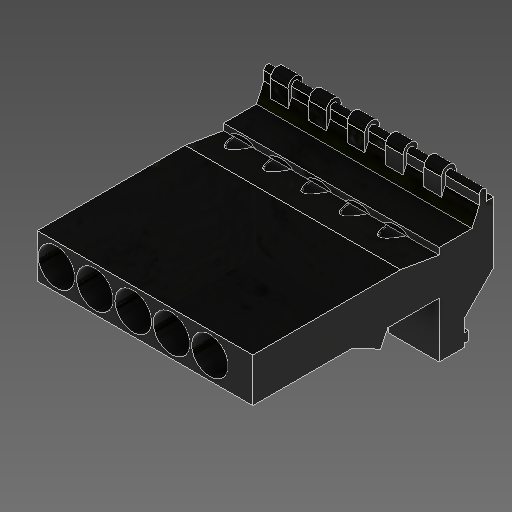
# Autodesk Inventor part: PostValveLast0
Saved by Autodesk Inventor 2020 (Build 240168000, 168)
## iProperties
Created: 2018-10-10
Part Number: PostValveLast0
Material: PLA Plastic (Black)
Document SubType Name: Modeling
Designer: Isaac Newcomb
Density: 1.06 g/cm^3
Appearance: 3D Printed - Black
Mass: 35.4889 g
Surface Area: 271.602 cm^2
Volume: 33.4801 cm^3
HingeHeight: 7.000 mm
KeyWidth: 10.000 mm
WhistleHousingHeight: 12.000 mm
PVBoxHeight: 20.163 mm
WhistleHousingLength: 51.000 mm
PVBoxDepth: 15.000 mm
HingeRadius: 1.000 mm
HingeOffset: 2.000 mm
HingeBigRadius: 2.000 mm
HingeBlockHeight: 4.500 mm
TubeSocketLength: 10.000 mm
SiliconeFittingLength: 10.000 mm
KeyCount: 25.000 ul
KeySpacing: 0.500 mm
SpringBlockHeight: 7.000 mm
SpringPassChamferLength: 8.000 mm
PincherTriangleHeight: 4.081 mm
PincherTriangleOffset: 31.000 mm
ManifoldWidth: 15.000 mm
ManifoldFittingLength: 10.000 mm
WhistleHousingVertWallThickness: 1.400 mm
Author: Isaac Newcomb
Autodesk Inventor part; units mm, degrees
ref_plane "YZ Plane" through (0, 0, 0) normal (1, 0, 0) x (0, 1, 0)
ref_plane "XZ Plane" through (0, 0, 0) normal (0, 1, 0) x (-1, 0, 0)
ref_plane "XY Plane" through (0, 0, 0) normal (0, 0, 1) x (1, 0, 0)
sketch "Base Sketch" plane through (0, 0, 0) normal (0, 0, 1) x (1, 0, 0)
  line L0 (0, 0) -> (10.5, 0)
  line L1 (10.5, 0) -> (10.5, 20.1625)
  line L2 (10.5, 20.1625) -> (0, 20.1625)
  line L3 (0, 20.1625) -> (0, 0)
  line L4 (1, 19.1625) -> (9.5, 19.1625)
  line L5 (9.5, 19.1625) -> (9.5, 1)
  line L6 (9.5, 1) -> (1, 1)
  line L7 (1, 1) -> (1, 19.1625)
  dimension "PVBoxWidth" = 10.5
  dimension "PVBoxHeight" = 20.1625
  dimension "SideWallThickness" = 1
  constraints: 16 end point, 4 parallel, 2 perpendicular, 1 horizontal, 3 other
  measures "PVBoxWidth" distance of L2.end L1.end
  measures "PVBoxHeight" distance of L2.end L0.start
  measures "SideWallThickness" distance between parallel lines of L2 L4
extrude "Side Walls" add sketch "Base Sketch" along normal blind 15
extrude "Back Wall" add sketch "Base Sketch" along normal blind 1 contours L4 L5 L6 L7
sketch "Sketch5" plane through (0, 0, 15) normal (0, 0, 1) x (1, 0, 0)
  line L0 (1, 19.1625) -> (9.5, 19.1625) projected
  line L1 (1, 1) -> (1, 19.1625) projected
  line L2 (9.5, 1) -> (1, 1) projected
  line L3 (9.5, 19.1625) -> (9.5, 1) projected
  point P0 (0, 0)
extrude "Front Wall" add sketch "Sketch5" against normal blind 5
sketch "Whistle Housing Sketch" plane through (0, 0, 15) normal (0, 0, 1) x (1, 0, 0)
  line L0 (0, 0) -> (10.5, 0) projected
  line L1 (0, 0) -> (0, 12)
  line L2 (0, 12) -> (10.5, 12)
  line L3 (10.5, 12) -> (10.5, 0)
  circle A0 centre (5.25, 6) radius 4.6
  line L4 (0, 6) -> (10.5, 6) construction
  line L5 (0, 12) -> (10.5, 12)
  line L6 (10.5, 12) -> (10.5, 15.5)
  line L7 (10.5, 15.5) -> (0, 15.5)
  line L8 (0, 15.5) -> (0, 12)
  dimension "WhistleHousingHeight" = 12
  dimension "TubeInnerDiameter" = 9.2
  dimension "TabThickness" = 3.5
  constraints: 16 end point, 3 midpoint, 3 perpendicular, 2 parallel, 1 centre point, 1 coincident, 1 horizontal, 1 vertical
  measures "WhistleHousingHeight" distance of L0.start L1.end
  measures "TubeInnerDiameter" diameter of A0
  measures "TabThickness" distance of L7.end L1.end
extrude "Whistle Housing" add sketch "Whistle Housing Sketch" along normal blind 51 contours L1 L2 L3 L0
sketch "Tube Socket Sketch" plane through (0, 0, 66) normal (0, 0, 1) x (1, 0, 0)
  circle A0 centre (5.25, 6) radius 4.6 construction
  circle A1 centre (5.25, 6) radius 5
  point P0 (0, 0)
  dimension "d78" = 10
  constraints: 1 centre point, 1 coincident
  measures "d78" diameter of A1
extrude "Tube Socket" cut sketch "Tube Socket Sketch" against normal blind 10
ref_plane "Midplane" through (5.25, 0, 0) normal (1, 0, 0) x (0, 0, -1)
sketch "Slit Sketch" plane through (0, 0, 15) normal (0, 0, 1) x (1, 0, 0)
  arc A0 (1.6989, 1.8) -> (8.8011, 1.8) centre (5.25, 6) ccw
  line L0 (8.8011, 1.8) -> (1.6989, 1.8)
  point P0 (0, 0)
  dimension "d81" = 11
  dimension "d187" = 5.25
  dimension "d188" = 6
  dimension "d193" = 4.2
  dimension "d194" = 1.3
  constraints: 2 end point, 2 point on circle, 1 centre point, 1 horizontal
  measures "d81" diameter of A0
  measures "d187" horizontal distance of point (0, 0) A0.centre
  measures "d188" vertical distance of point (0, 0) A0.centre
  measures "d193" distance from line of L0 A0.centre
  measures "d194" distance edge to line of A0 L0
extrude "Slit" cut sketch "Slit Sketch" against normal up to surface (14 mm away)
sketch "Silicone Fitting Sketch" plane through (5.25, 0, 0) normal (1, 0, 0) x (0, 0, -1)
  line L0 (-15, 20.1625) -> (-15, 12) projected
  line L1 (-15, 16.0813) -> (-25, 16.0813) construction
  line L2 (-25, 16.0813) -> (-25, 18.4625)
  line L3 (-25, 18.4625) -> (-22, 18.4625) construction
  line L4 (-25, 18.4625) -> (-22, 19.1625)
  line L5 (-22, 19.1625) -> (-22, 18.4625)
  line L6 (-25, 17.9625) -> (-15, 17.9625)
  line L7 (-22, 18.4625) -> (-19, 18.4625) construction
  line L8 (-15, 19.1625) -> (-22, 19.1625) construction
  line L9 (-22, 18.4625) -> (-19, 19.1625)
  line L10 (-19, 19.1625) -> (-19, 18.4625)
  line L11 (-19, 18.4625) -> (-15, 18.4625)
  point P0 (0, 0)
  point P1 (-15, 0)
  dimension "SiliconeFittingLength" = 10
  dimension "d65" = 2.3813
  dimension "d66" = 3
  dimension "d67" = 0.7
  dimension "d68" = 0.5
  constraints: 22 end point, 10 perpendicular, 5 point on line, 4 parallel, 2 horizontal, 2 midpoint
  measures "SiliconeFittingLength" distance of L1.start L1.end
  measures "d65" distance of L1.end L2.end
  measures "d66" horizontal distance of L4.end L2.end
  measures "d67" distance of L4.end L3.end
  measures "d68" distance between parallel lines of L3 L6
revolve "Silicone Fitting" add sketch "Silicone Fitting Sketch" angle 360 about axis through (5.25, 16.0813, 15) along (0, 0, 1)
sketch "Silicone Fitting to Chamber Sketch" plane through (5.25, 16.0813, 15) normal (0, 0, 1) x (1, 0, 0)
  circle A0 centre (0, 0) radius 1.8813 projected
  point P0 (-5.25, -16.0813)
extrude "Silicone Fitting to Chamber" cut sketch "Silicone Fitting to Chamber Sketch" against normal up to surface (5 mm away)
sketch "Hinge Sketch" plane through (10.5, 0, 0) normal (1, 0, 0) x (0, 0, -1)
  line L0 (0, 0) -> (-66, 0) projected
  line L1 (-2, 0) -> (-2, -4.5) construction
  arc A0 (-4, -7) -> (-2, -7) centre (-3, -7) ccw
  line L2 (-4, -7) -> (-4, -4.5)
  line L3 (-2, -4.5) -> (0, -4.5)
  line L4 (0, -4.5) -> (0, 0)
  line L5 (-4, -4.5) -> (-6, -4.5)
  line L6 (-6, -4.5) -> (-6, 0)
  line L7 (-2, -4.5) -> (-2, -7)
  line L8 (-4, -4.5) -> (-4, 0) construction
  point P0 (-15, 0)
  dimension "HingeRadius" = 1
  dimension "HingeBlockHeight" = 4.5
  dimension "HingeOffset" = 2
  dimension "HingeHeight" = 7
  constraints: 16 end point, 5 point on line, 4 perpendicular, 4 tangent, 2 point on circle, 2 vertical, 1 centre point, 1 collinear, 1 horizontal
  measures "HingeRadius" radius of A0
  measures "HingeBlockHeight" distance of L3.end L0.start
  measures "HingeOffset" distance of L1.end L3.end
  measures "HingeHeight" distance from line of L0 A0.centre
extrude "Hinge" add sketch "Hinge Sketch" against normal blind 10.5
sketch "Hinge Nub Sketch" plane through (5.25, 20.1625, 15) normal (1, 0, 0) x (0, 0, -1)
  arc A0 (11, -27.1625) -> (13, -27.1625) centre (12, -27.1625) ccw construction
  arc A1 (10, -27.1625) -> (14, -27.1625) centre (12, -27.1625) ccw
  line L0 (14, -27.1625) -> (14, -24.6625)
  line L1 (15, -24.6625) -> (9, -24.6625)
  line L2 (10, -24.6625) -> (10, -27.1625)
  point P0 (15, -20.1625)
  point P1 (9, -20.1625)
  dimension "HingeBigRadius" = 2
  constraints: 6 end point, 2 point on circle, 2 point on line, 2 tangent, 1 centre point, 1 coincident, 1 parallel, 1 perpendicular, 1 vertical
  measures "HingeBigRadius" radius of A1
extrude "Hinge Nub" add sketch "Hinge Nub Sketch" along normal mid plane 4.8
chamfer "Hinge Clearance Chamfer" distance 2 distance2 4.5 1 edges at (5.25, -4.5, 6) measured on face at (5.25, -4.5, 5.5)
chamfer "Spring Pass Chamfer" distance 8 angle 45 2 edges at (5.25, 19.1625, 1) (5.25, 20.1625, 0)
sketch "Spring Block Sketch" plane through (0, 20.1625, 15) normal (0, 1, 0) x (1, 0, 0)
  line L0 (7.35, 7) -> (2.1, 7)
  line L1 (2.1, 7) -> (2.1, 0)
  line L2 (2.1, 0) -> (7.35, 0)
  line L3 (7.35, 0) -> (7.35, 7)
  point P0 (0, 15)
  point P1 (0, 15)
  dimension "d135" = 5.25
  dimension "d136" = 8
  dimension "d137" = 15
  dimension "d289" = 2.1
  constraints: 8 end point, 2 parallel, 1 coincident, 1 horizontal, 1 perpendicular
  measures "d135" distance of L0.start L0.end
  measures "d136" distance from line of point (0, 15) L0
  measures "d137" distance from line of point (0, 15) L2
  measures "d289" distance from line of point (0, 15) L1
extrude "Spring Block" add sketch "Spring Block Sketch" along normal blind 7
sketch "Spring Hook Sketch" plane through (7.35, 20.1625, 15) normal (1, 0, 0) x (0, 0, -1)
  line L0 (8, 3.5) -> (5, 3.5)
  line L1 (5, 3.5) -> (5, 6)
  line L2 (5, 6) -> (8, 6)
  line L3 (8, 6) -> (8, 3.5)
  point P0 (15, -20.1625)
  dimension "d160" = 3
  dimension "d161" = 2.5
  dimension "d162" = 10
  dimension "d171" = 26.1625
  constraints: 8 end point, 2 parallel, 1 horizontal, 1 perpendicular
  measures "d160" distance of L1.end L2.end
  measures "d161" distance of L0.end L1.end
  measures "d162" distance from line of point (15, -20.163) L1
  measures "d171" distance from line of L2 point (15, -20.163)
extrude "Spring Hook" add sketch "Spring Hook Sketch" along normal blind 4 and the other way blind 5.25
draft "Sping Hook Draft" angle 20 pull direction (-1, 0, 0) faces at (10.0167, 25.3292, 10) fixed edges at (11.35, 24.9125, 10)
fillet "Spring Hook Fillet" radius 1 3 edges at (9.35, 23.6625, 9.2721) (9.35, 26.1625, 9.2721) (7.35, 24.9125, 8.5441)
sketch "Edge Cut Sketch" plane through (5.25, 0, 0) normal (1, 0, 0) x (0, 0, -1)
  line L0 (-15, 1.4) -> (-15, 0)
  line L1 (-25.5368, 0) -> (-15, 1.8)
  line L2 (-15, 1.4) -> (-15, 1.8)
  line L3 (-15, 1.4) -> (-19.7, 1.4) construction
  arc A0 (-19.6663, 1.0029) -> (-19.7, 1.4) centre (-19.7, 1.2) ccw construction
  line L4 (-19.5, 1.4) -> (-19.5, 1.0313) construction
  line L5 (-15, 0) -> (-25.5368, 0)
  point P0 (0, 0)
  dimension "EdgeCutDepth" = 0.4
  dimension "d101" = 0.2
  dimension "EdgeDistance" = 4.5
  dimension "d190" = 15
  dimension "d191" = 0
  dimension "WhistleHousingVertWallThickness" = 1.4
  constraints: 13 end point, 3 point on line, 3 tangent, 2 point on circle, 2 vertical, 1 centre point, 1 collinear, 1 horizontal, 1 perpendicular
  measures "EdgeCutDepth" distance of L0.start L1.end
  measures "d101" radius of A0
  measures "EdgeDistance" distance between parallel lines of L0 L4
  measures "d190" distance of point (0, 0) L0.end
  measures "d191" vertical distance of point (0, 0) L0.end
  measures "WhistleHousingVertWallThickness" distance of L0.start L0.end
extrude "Edge Cut" cut sketch "Edge Cut Sketch" along normal mid plane 10.5
fillet "Edge Fillet" radius 0.2 1 edges at (5.25, 1.4, 17.3415)
sketch "Pincher Triangle Sketch" plane through (5.25, 0, 0) normal (1, 0, 0) x (0, 0, -1)
  line L0 (-29, 12) -> (-39, 12)
  line L1 (-39, 12) -> (-31, 16.0813)
  line L2 (-31, 16.0813) -> (-29, 12)
  line L3 (-31, 16.0813) -> (-31, 12) construction
  line L4 (-36.7995, 12) -> (-31.4508, 14.7287)
  line L5 (-31.4508, 14.7287) -> (-30.1136, 12)
  line L6 (-30.3363, 12) -> (-31.5409, 14.4581)
  line L7 (-31.5409, 14.4581) -> (-36.3594, 12)
  point P0 (0, 0)
  dimension "PincherTriangleHeight" = 4.0812
  dimension "d173" = 12
  dimension "PincherTriangleOffset" = 31
  dimension "d284" = 1
  dimension "d285" = 0.2
  dimension "d304" = 2
  dimension "d305" = 8
  dimension "d306" = 0.2
  dimension "d307" = 1
  constraints: 16 end point, 5 point on line, 4 parallel, 1 horizontal, 1 perpendicular
  measures "PincherTriangleHeight" distance of L1.end L3.end
  measures "d173" vertical distance of point (0, 0) L0.start
  measures "PincherTriangleOffset" distance from line of point (0, 0) L3
  measures "d284" distance between parallel lines of L2 L5
  measures "d285" distance between parallel lines of L5 L6
  measures "d304" distance from line of L3 L0.start
  measures "d305" distance from line of L3 L0.end
  measures "d306" distance between parallel lines of L7 L4
  measures "d307" distance between parallel lines of L4 L1
extrude "Pincher Triangle" add sketch "Pincher Triangle Sketch" along normal mid plane 10.5 contours L0 L5 L4 L1 L2 | L0 L6 L7 L4 L5
extrude "Triangle Coupling Male" add sketch "Pincher Triangle Sketch" along normal blind 10.5 contours L0 L7 L6
extrude "Fill: Triangle Coupling Female" add sketch "Pincher Triangle Sketch" against normal blind 5.25 contours L0 L7 L6
pattern_linear "Key Repitition" count 5 spacing 10.5 along (-1, 0, 0)
sketch "Sketch28" plane through (-42, -4.5, 0) normal (-1, 0, 0) x (0, 0, 1)
  line L0 (39, 16.5) -> (31, 20.5813) projected
  line L1 (31, 20.5813) -> (29, 16.5) projected
  line L2 (15, 16.5) -> (29, 16.5) projected
  line L3 (15, 24.6625) -> (15, 16.5) projected
  line L4 (8, 24.6625) -> (15, 24.6625) projected
  line L5 (0, 16.6625) -> (8, 24.6625) projected
  line L6 (0, 16.6625) -> (0, 0) projected
  line L7 (0, 0) -> (2, 0) projected
  line L8 (2, 0) -> (2, -2.5) projected
  arc A0 (2, -2.5) -> (4, -2.5) centre (3, -2.5) ccw projected
  line L9 (4, -2.5) -> (4, 0) projected
  line L10 (6, 4.5) -> (4, 0) projected
  line L11 (6, 4.5) -> (15, 4.5) projected
  line L12 (15, 4.5) -> (15, 6.3) projected
  line L13 (15, 6.3) -> (25.5368, 4.5) projected
  line L14 (25.5368, 4.5) -> (66, 4.5) projected
  line L15 (66, 16.5) -> (66, 4.5) projected
  line L16 (39, 16.5) -> (66, 16.5) projected
  point P0 (0, 4.5)
extrude "Extrusion28" add sketch "Sketch28" along normal blind 6.5
sketch "Sketch29" plane through (-39.9, 20.1625, 15) normal (-1, 0, 0) x (0, 0, 1)
  line L0 (-7, 0) -> (-7, 3.5) projected
  line L1 (0, 0) -> (-7, 0) projected
  line L2 (0, 0) -> (0, 7) projected
  line L3 (-7, 7) -> (0, 7) projected
  line L4 (-7, 6) -> (-7, 7) projected
  line L5 (-7, 6) -> (-8, 6) projected
  line L6 (-8, 6) -> (-8, 3.5) projected
  line L7 (-8, 3.5) -> (-7, 3.5) projected
  point P0 (-15, -20.1625)
extrude "Extrusion29" add sketch "Sketch29" along normal up to surface (8.6 mm away)
fillet "Fillet20" radius 0.4 6 edges at (13.125, 12, 36.3594) (13.125, 12, 30.3363) (15.75, 12, 33.3479) (15.75, 13.2291, 33.9502) (13.125, 14.4581, 31.5409) (15.75, 13.2291, 30.9386)
equation "\"PVBoxWidth\" = KeyWidth + KeySpacing"
equation "\"SideWallThickness\" = WallThickness"
equation "\"BackWallThickness\" = WallThickness"
equation "\"TubeInnerDiameter\" = KeyWidth - 2 * TubeWallThickness"
equation "\"d88\" = KeySpacing + KeyWidth"
equation "\"EdgeCutDepth\" = TubeWallThickness"
equation "\"KeyCount\" = 25"
equation "\"KeyWidth\" = 10"
equation "\"KeySpacing\" = 0.5"
equation "\"WallThickness\" = 1"
equation "\"TubeWallThickness\" = 0.4"
equation "\"ManifoldWidth\" = 15"
equation "\"ManifoldFittingLength\" = 10"
equation "\"WhiteKeyWidth\" = 17.5"
equation "\"TopCKeyRightWidth\" = 11.75"
body "Solid1"
